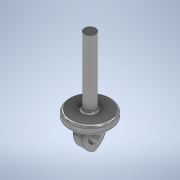
# Autodesk Inventor part: Part4
Saved by Autodesk Inventor 2020 (Build 240168000, 168)
## iProperties
Created: 2021-05-18
Part Number: Part4
Material: Aluminum 6061
Document SubType Name: Modeling
Designer: Andrew
Density: 2.7 g/cm^3
Appearance: Chrome - Polished Black
Mass: 332.111 g
Surface Area: 234.486 cm^2
Volume: 123.004 cm^3
Author: Andrew
Autodesk Inventor part; units mm, degrees
ref_plane "YZ Plane" through (0, 0, 0) normal (1, 0, 0) x (0, 1, 0)
ref_plane "XZ Plane" through (0, 0, 0) normal (0, 1, 0) x (-1, 0, 0)
ref_plane "XY Plane" through (0, 0, 0) normal (0, 0, 1) x (1, 0, 0)
sketch "Sketch1" plane through (0, 0, 0) normal (1, 0, 0) x (0, 1, 0)
  line L0 (0, 0) -> (0, -9.85)
  line L1 (0, -9.85) -> (-120, -9.85)
  line L2 (-120, -9.85) -> (-120, -37.5)
  line L3 (-120, -37.5) -> (-135, -37.5)
  line L4 (-135, -37.5) -> (-135, 0)
  line L5 (-135, 0) -> (0, 0)
  line L6 (-135, 0) -> (-135, 22.5)
  line L7 (-135, 22.5) -> (-150, 22.5)
  line L8 (-135, 0) -> (-135, -22.5)
  line L9 (-135, -22.5) -> (-150, -22.5)
  arc A0 (-150, 22.5) -> (-181.8198, 0) centre (-150, -11.25) ccw
  arc A1 (-181.8198, 0) -> (-150, -22.5) centre (-150, 11.25) ccw
  arc A2 (-120, -10.1) -> (-119.8236, -9.85) centre (-150, 11.25) ccw
  circle A3 centre (-160, 0) radius 10
  dimension "d0" = 9.85
  dimension "d1" = 120
  dimension "d2" = 27.65
  dimension "d3" = 15
  dimension "d4" = 22.5
  dimension "d5" = 15
  dimension "d6" = 22.5
  dimension "d14" = 33.75
  dimension "d15" = 33.75
  dimension "d16" = 20
  dimension "d17" = 25
  constraints: 20 end point, 6 perpendicular, 6 point on circle, 4 centre point, 3 point on line, 2 vertical, 1 parallel
  measures "d0" distance of L0.start L0.end
  measures "d1" distance of L0.end L1.end
  measures "d2" distance of L1.end L2.end
  measures "d3" distance of L2.end L3.end
  measures "d4" distance of L4.end L6.end
  measures "d5" distance of L7.end L6.end
  measures "d6" distance of L4.end L8.end
  measures "d14" radius of A1
  measures "d15" radius of A0
  measures "d16" diameter of A3
  measures "d17" distance of A3.centre L4.end
revolve "Revolution1" add sketch "Sketch1" angle 360 about axis through (0, -135, 0) along (0, 1, 0) contours L0 L1 L2 L3 L4 L5
extrude "Extrusion1" add sketch "Sketch1" along normal mid plane 15 contours L4 L9 A1 A0 L7 L6
fillet "Fillet1" radius 4 7 edges at (0, -120, 37.5) (0, -135, 37.5) (0, -120, 9.85) (7.5, -135, 0) (0, -135, 22.5) (0, -135, -22.5) (-7.5, -135, 0)
fillet "Fillet2" radius 4 1 edges at (0, -181.8198, 0)
body "Solid1"
